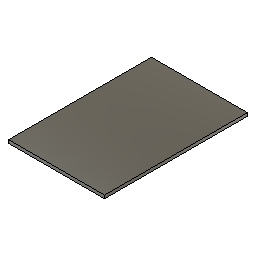
Spray Base (Autodesk Fusion 360 archive; units mm, degrees)
design "spraytest" references "autodesk generic router xyz"
Autodesk Fusion 360 part; units mm, degrees
sketch "Sketch1" plane through (0, 0, 0) normal (0, 0, 1) x (1, 0, 0)
  line L0 (571.5, 850.9) -> (-571.5, 850.9)
  line L1 (-571.5, 850.9) -> (-571.5, -850.9)
  line L2 (-571.5, -850.9) -> (571.5, -850.9)
  line L3 (571.5, -850.9) -> (571.5, 850.9)
  line L4 (571.5, 850.9) -> (-571.5, -850.9) construction
  line L5 (-571.5, 850.9) -> (571.5, -850.9) construction
  dimension "d1" = 1143
  dimension "d2" = 1701.8
  constraint horizontal L0
  constraint perpendicular L0 L1
  constraint parallel L0 L2
  constraint parallel L1 L3
  constraint coincident L4 origin
  constraint coincident L5 origin
  measures "d1" distance of L1.end L2.end
  measures "d2" distance of L0.end L1.end
extrude "Extrude1" add sketch "Sketch1" along normal blind 38.1
equation "d2 = 134 in / 2"
